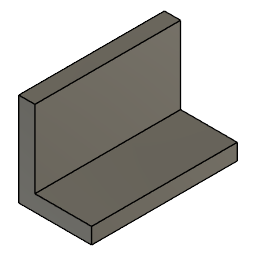
Ex2-lab1 (Autodesk Fusion 360 design; units mm, degrees)
part number: 2026-03-02-19-41-34-986
Autodesk Fusion 360 part; units mm, degrees
sketch "Sketch1" plane through (0, 0, 0) normal (0, 0, 1) x (1, 0, 0)
  line L0 (-36.2598, 58.769) -> (-36.2598, 0)
  line L1 (-36.2598, 0) -> (8.7402, 0)
  line L2 (8.7402, 0) -> (8.7402, 10)
  line L3 (-36.2598, 58.769) -> (-26.2598, 58.769)
  line L4 (-26.2598, 58.769) -> (-26.2598, 10)
  line L5 (-26.2598, 10) -> (8.7402, 10)
  dimension "d1" = 45
  dimension "d2" = 10
  dimension "d3" = 10
  constraint vertical L0
  constraint perpendicular L0 L1
  constraint perpendicular L1 L2
  constraint perpendicular L0 L3
  constraint perpendicular L3 L4
  constraint perpendicular L2 L5
  measures "d1" distance of L0.end L1.end
  measures "d2" distance of L1.end L2.end
  measures "d3" distance of L0.start L3.end
extrude "Extrude1" add sketch "Sketch1" along normal blind 90
sketch "Sketch2" plane through (0, 0, 0) normal (0, 0, 1) x (1, 0, 0)
move_body "Move1" bodies 1 to x (1, 0, 0) y (0, 0, 1) z (0, -1, 0) at (0, 103.769, -13.769)
move_body "Move2" bodies 1 to x (1, 0, 0) y (0, 1, 0) z (0, 0, 1) at (0, 0, 10)
move_body "Move3" bodies 1 to x (1, 0, 0) y (0, 1, 0) z (0, 0, 1) at (0, 0, 3)
move_face "MoveFace1" by (0, 0, 1) 3 faces at (-14.5931, 73.769, 9.231) (8.7402, 43.769, 5.8977) (-21.2598, 73.769, -0.769)
